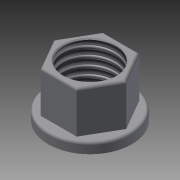
# Autodesk Inventor part: 刀夹片紧固螺帽
Saved by Autodesk Inventor 2015 (Build 190159000, 159)
## iProperties
Created: 2017-05-17
Part Number: 刀夹片紧固螺帽
Material: 常规
Document SubType Name: Modeling
Designer: Administrator
Density: 1 g/cm^3
Appearance: 默认
Author: Administrator
Autodesk Inventor part; units mm, degrees
ref_plane "YZ Plane" through (0, 0, 0) normal (1, 0, 0) x (0, 1, 0)
ref_plane "XZ Plane" through (0, 0, 0) normal (0, 1, 0) x (-1, 0, 0)
ref_plane "XY Plane" through (0, 0, 0) normal (0, 0, 1) x (1, 0, 0)
sketch "草图1" plane through (0, 0, 0) normal (0, 0, 1) x (1, 0, 0)
  circle A0 centre (0, 0) radius 4
  dimension "d0" = 8
  constraints: 1 centre point, 1 coincident
  measures "d0" diameter of A0
extrude "拉伸1" add sketch "草图1" along normal blind 1
sketch "草图2" plane through (0, 0, 1) normal (0, 0, 1) x (1, 0, 0)
  line L0 (1.7321, -3) -> (-1.7321, -3)
  line L1 (-1.7321, -3) -> (-3.4641, 0)
  line L2 (-3.4641, 0) -> (-1.7321, 3)
  line L3 (-1.7321, 3) -> (1.7321, 3)
  line L4 (1.7321, 3) -> (3.4641, 0)
  line L5 (3.4641, 0) -> (1.7321, -3)
  line L6 (0, 0) -> (0, 0.9644)
  point P0 (0, 3)
  dimension "d3" = 0.9644
  dimension "d4" = 6
  constraints: 14 end point, 1 coincident, 1 midpoint, 1 point on line, 1 vertical, 13 other
  measures "d3" distance of L6.start L6.end
  measures "d4" distance between parallel lines of L0 L3
extrude "拉伸2" add sketch "草图2" along normal blind 4
sketch "草图3" plane through (0, 0, 5) normal (0, 0, 1) x (1, 0, 0)
  circle A0 centre (0, 0) radius 2.5
  dimension "d7" = 5
  constraints: 1 centre point, 1 coincident
  measures "d7" diameter of A0
extrude "拉伸3" cut sketch "草图3" against normal through all
thread "螺纹1" size "M5x0.8" class "6H" standard "ANSI Metric M Profile" full length
fillet "圆角1" radius 0.25 7 edges at (-2.5981, 1.5, 5) (-2.5981, -1.5, 5) (0, 3, 5) (2.5981, 1.5, 5) (2.5981, -1.5, 5) (0, -3, 5) (-4, 0, 1)
chamfer "倒角1" distance 0.1 angle 45 1 edges at (-2.5, 0, 5)
